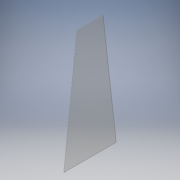
# Autodesk Inventor part: Polycarb Back Pannel
Saved by Autodesk Inventor 2016 (Build 200138000, 138)
## iProperties
Created: 2018-05-16
Part Number: Polycarb Back Pannel
Material: Polycarbonate, Clear
Document SubType Name: Modeling
Designer: Kade
Density: 1.2 g/cm^3
Appearance: Polycarbonate - Clear
Mass: 1068.25 g
Surface Area: 5685.53 cm^2
Volume: 890.211 cm^3
Author: Kade
Autodesk Inventor part; units mm, degrees
ref_plane "YZ Plane" through (0, 0, 0) normal (1, 0, 0) x (0, 1, 0)
ref_plane "XZ Plane" through (0, 0, 0) normal (0, 1, 0) x (-1, 0, 0)
ref_plane "XY Plane" through (0, 0, 0) normal (0, 0, 1) x (1, 0, 0)
sketch "Sketch1" plane through (0, 0, 0) normal (1, 0, 0) x (0, 1, 0)
  line L0 (0, 0) -> (0, 410.0576)
  line L1 (0, 0) -> (0, 205.0288)
  line L2 (0, 205.0288) -> (914.4, 205.0288) construction
  line L3 (914.4, 306.6288) -> (914.4, 103.4288)
  line L4 (914.4, 306.6288) -> (0, 410.0576)
  line L5 (914.4, 103.4288) -> (0, 0)
  dimension "d0" = 410.0576
  dimension "d2" = 914.4
  dimension "d4" = 203.2
  dimension "d5" = 205.0288
  dimension "d6" = 920.2309
  dimension "d7" = 920.2309
  constraints: 12 end point, 1 horizontal, 1 midpoint, 1 parallel, 1 vertical
  measures "d0" distance of L0.start L0.end
  measures "d2" distance of L1.end L2.end
  measures "d4" distance of L3.start L3.end
  measures "d5" distance from line of L0.start L2
  measures "d6" distance of L3.start L0.end
  measures "d7" distance of L3.end L0.start
extrude "Extrusion1" add sketch "Sketch1" along normal blind 3.175
body "Solid1"
